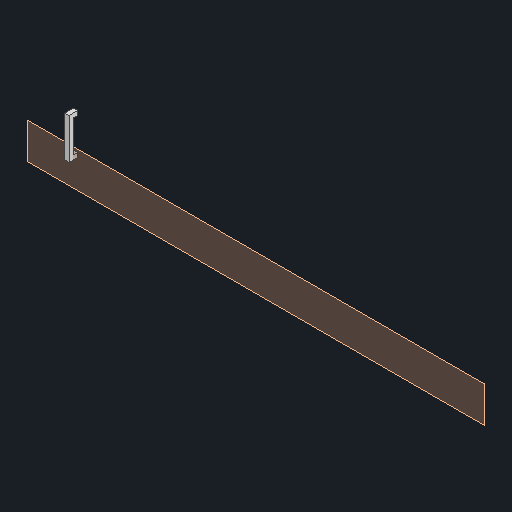
# Autodesk Inventor part: Reinforcer
Saved by Autodesk Inventor 2027 (Build 310192000, 192)
## iProperties
Created: 2026-04-15
Part Number: Reinforcer
Material: Generic
Document SubType Name: Modeling
Designer: Tueha
Density: 1 g/cm^3
Appearance: Default
Author: Tueha
Autodesk Inventor part; units mm, degrees
ref_plane "YZ Plane" through (0, 0, 0) normal (1, 0, 0) x (0, 1, 0)
ref_plane "XZ Plane" through (0, 0, 0) normal (0, 1, 0) x (-1, 0, 0)
ref_plane "XY Plane" through (0, 0, 0) normal (0, 0, 1) x (1, 0, 0)
ref_plane "Work Plane1" through (504.7277, -38.7707, -20.8442) normal (0, 0, 1) x (-1, 0, 0)
sketch "Sketch1" plane through (504.7277, -38.7707, -20.8442) normal (0, 0, 1) x (-1, 0, 0)
  line L0 (-28.8, -55.1) -> (-22.6, -55.1) projected
  line L1 (-28.8, -72) -> (-28.8, -55.1) projected
  line L2 (-28.8, -72) -> (262.8, -72) projected
  line L3 (262.8, -72) -> (262.8, -78) projected
  line L4 (262.8, -78) -> (-28.8, -78) projected
  line L5 (-28.8, -94.9) -> (-28.8, -78) projected
  line L6 (-13.3962, -94.9) -> (-28.8, -94.9) projected
  line L7 (-8.2, -97.9) -> (-13.3962, -94.9) projected
  line L8 (-8.2, -94.9) -> (-8.2, -97.9) projected
  arc A0 (-6.2, -94.9) -> (-8.2, -94.9) centre (-7.2, -94.9) ccw projected
  line L9 (-6.2, -97.9) -> (-6.2, -94.9) projected
  line L10 (-1.0038, -94.9) -> (-6.2, -97.9) projected
  line L11 (15.4038, -94.9) -> (-1.0038, -94.9) projected
  line L12 (20.6, -97.9) -> (15.4038, -94.9) projected
  line L13 (20.6, -94.9) -> (20.6, -97.9) projected
  arc A1 (22.6, -94.9) -> (20.6, -94.9) centre (21.6, -94.9) ccw projected
  line L14 (22.6, -97.9) -> (22.6, -94.9) projected
  line L15 (27.7962, -94.9) -> (22.6, -97.9) projected
  line L16 (44.2038, -94.9) -> (27.7962, -94.9) projected
  line L17 (49.4, -97.9) -> (44.2038, -94.9) projected
  line L18 (49.4, -94.9) -> (49.4, -97.9) projected
  arc A2 (51.4, -94.9) -> (49.4, -94.9) centre (50.4, -94.9) ccw projected
  line L19 (51.4, -97.9) -> (51.4, -94.9) projected
  line L20 (56.5962, -94.9) -> (51.4, -97.9) projected
  line L21 (73.0038, -94.9) -> (56.5962, -94.9) projected
  line L22 (78.2, -97.9) -> (73.0038, -94.9) projected
  line L23 (78.2, -94.9) -> (78.2, -97.9) projected
  arc A3 (80.2, -94.9) -> (78.2, -94.9) centre (79.2, -94.9) ccw projected
  line L24 (80.2, -97.9) -> (80.2, -94.9) projected
  line L25 (85.3962, -94.9) -> (80.2, -97.9) projected
  line L26 (101.8038, -94.9) -> (85.3962, -94.9) projected
  line L27 (107, -97.9) -> (101.8038, -94.9) projected
  line L28 (107, -94.9) -> (107, -97.9) projected
  arc A4 (109, -94.9) -> (107, -94.9) centre (108, -94.9) ccw projected
  line L29 (109, -97.9) -> (109, -94.9) projected
  line L30 (114.1962, -94.9) -> (109, -97.9) projected
  line L31 (130.6038, -94.9) -> (114.1962, -94.9) projected
  line L32 (135.8, -97.9) -> (130.6038, -94.9) projected
  line L33 (135.8, -94.9) -> (135.8, -97.9) projected
  arc A5 (137.8, -94.9) -> (135.8, -94.9) centre (136.8, -94.9) ccw projected
  line L34 (137.8, -97.9) -> (137.8, -94.9) projected
  line L35 (142.9962, -94.9) -> (137.8, -97.9) projected
  line L36 (159.4038, -94.9) -> (142.9962, -94.9) projected
  line L37 (164.6, -97.9) -> (159.4038, -94.9) projected
  line L38 (164.6, -94.9) -> (164.6, -97.9) projected
  arc A6 (166.6, -94.9) -> (164.6, -94.9) centre (165.6, -94.9) ccw projected
  line L39 (166.6, -97.9) -> (166.6, -94.9) projected
  line L40 (171.7962, -94.9) -> (166.6, -97.9) projected
  line L41 (188.2038, -94.9) -> (171.7962, -94.9) projected
  line L42 (193.4, -97.9) -> (188.2038, -94.9) projected
  line L43 (193.4, -94.9) -> (193.4, -97.9) projected
  arc A7 (195.4, -94.9) -> (193.4, -94.9) centre (194.4, -94.9) ccw projected
  line L44 (195.4, -97.9) -> (195.4, -94.9) projected
  line L45 (200.5962, -94.9) -> (195.4, -97.9) projected
  line L46 (217.0038, -94.9) -> (200.5962, -94.9) projected
  line L47 (222.2, -97.9) -> (217.0038, -94.9) projected
  line L48 (222.2, -94.9) -> (222.2, -97.9) projected
  arc A8 (224.2, -94.9) -> (222.2, -94.9) centre (223.2, -94.9) ccw projected
  line L49 (224.2, -97.9) -> (224.2, -94.9) projected
  line L50 (229.3962, -94.9) -> (224.2, -97.9) projected
  line L51 (245.8038, -94.9) -> (229.3962, -94.9) projected
  line L52 (251, -97.9) -> (245.8038, -94.9) projected
  line L53 (251, -94.9) -> (251, -97.9) projected
  arc A9 (253, -94.9) -> (251, -94.9) centre (252, -94.9) ccw projected
  line L54 (253, -97.9) -> (253, -94.9) projected
  line L55 (258.1962, -94.9) -> (253, -97.9) projected
  line L56 (274.6038, -94.9) -> (258.1962, -94.9) projected
  line L57 (279.8, -97.9) -> (274.6038, -94.9) projected
  line L58 (279.8, -94.9) -> (279.8, -97.9) projected
  arc A10 (281.8, -94.9) -> (279.8, -94.9) centre (280.8, -94.9) ccw projected
  line L59 (281.8, -97.9) -> (281.8, -94.9) projected
  line L60 (286.9962, -94.9) -> (281.8, -97.9) projected
  line L61 (303.4038, -94.9) -> (286.9962, -94.9) projected
  line L62 (308.6, -97.9) -> (303.4038, -94.9) projected
  line L63 (308.6, -94.9) -> (308.6, -97.9) projected
  arc A11 (310.6, -94.9) -> (308.6, -94.9) centre (309.6, -94.9) ccw projected
  line L64 (310.6, -97.9) -> (310.6, -94.9) projected
  line L65 (315.7962, -94.9) -> (310.6, -97.9) projected
  line L66 (332.2038, -94.9) -> (315.7962, -94.9) projected
  line L67 (337.4, -97.9) -> (332.2038, -94.9) projected
  line L68 (337.4, -94.9) -> (337.4, -97.9) projected
  arc A12 (339.4, -94.9) -> (337.4, -94.9) centre (338.4, -94.9) ccw projected
  line L69 (339.4, -97.9) -> (339.4, -94.9) projected
  line L70 (344.5962, -94.9) -> (339.4, -97.9) projected
  line L71 (361.0038, -94.9) -> (344.5962, -94.9) projected
  line L72 (366.2, -97.9) -> (361.0038, -94.9) projected
  line L73 (366.2, -94.9) -> (366.2, -97.9) projected
  arc A13 (368.2, -94.9) -> (366.2, -94.9) centre (367.2, -94.9) ccw projected
  line L74 (368.2, -97.9) -> (368.2, -94.9) projected
  line L75 (373.3962, -94.9) -> (368.2, -97.9) projected
  line L76 (389.8038, -94.9) -> (373.3962, -94.9) projected
  line L77 (395, -97.9) -> (389.8038, -94.9) projected
  line L78 (395, -94.9) -> (395, -97.9) projected
  arc A14 (397, -94.9) -> (395, -94.9) centre (396, -94.9) ccw projected
  line L79 (397, -97.9) -> (397, -94.9) projected
  line L80 (402.1962, -94.9) -> (397, -97.9) projected
  line L81 (418.6038, -94.9) -> (402.1962, -94.9) projected
  line L82 (423.8, -97.9) -> (418.6038, -94.9) projected
  line L83 (423.8, -94.9) -> (423.8, -97.9) projected
  arc A15 (425.8, -94.9) -> (423.8, -94.9) centre (424.8, -94.9) ccw projected
  line L84 (425.8, -97.9) -> (425.8, -94.9) projected
  line L85 (430.9962, -94.9) -> (425.8, -97.9) projected
  line L86 (447.4038, -94.9) -> (430.9962, -94.9) projected
  line L87 (452.6, -97.9) -> (447.4038, -94.9) projected
  line L88 (452.6, -94.9) -> (452.6, -97.9) projected
  arc A16 (454.6, -94.9) -> (452.6, -94.9) centre (453.6, -94.9) ccw projected
  line L89 (454.6, -97.9) -> (454.6, -94.9) projected
  line L90 (459.7962, -94.9) -> (454.6, -97.9) projected
  line L91 (476.2038, -94.9) -> (459.7962, -94.9) projected
  line L92 (481.4, -97.9) -> (476.2038, -94.9) projected
  line L93 (481.4, -94.9) -> (481.4, -97.9) projected
  arc A17 (483.4, -94.9) -> (481.4, -94.9) centre (482.4, -94.9) ccw projected
  line L94 (483.4, -97.9) -> (483.4, -94.9) projected
  line L95 (488.5962, -94.9) -> (483.4, -97.9) projected
  line L96 (505.0038, -94.9) -> (488.5962, -94.9) projected
  line L97 (510.2, -97.9) -> (505.0038, -94.9) projected
  line L98 (510.2, -94.9) -> (510.2, -97.9) projected
  arc A18 (512.2, -94.9) -> (510.2, -94.9) centre (511.2, -94.9) ccw projected
  line L99 (512.2, -97.9) -> (512.2, -94.9) projected
  line L100 (517.3962, -94.9) -> (512.2, -97.9) projected
  line L101 (533.8038, -94.9) -> (517.3962, -94.9) projected
  line L102 (539, -97.9) -> (533.8038, -94.9) projected
  line L103 (539, -94.9) -> (539, -97.9) projected
  arc A19 (541, -94.9) -> (539, -94.9) centre (540, -94.9) ccw projected
  line L104 (541, -97.9) -> (541, -94.9) projected
  line L105 (546.1962, -94.9) -> (541, -97.9) projected
  line L106 (546.1962, -94.9) -> (554.4, -94.9) projected
  line L107 (554.4, -55.1) -> (554.4, -94.9) projected
  line L108 (531.7962, -55.1) -> (554.4, -55.1) projected
  line L109 (526.6, -52.1) -> (531.7962, -55.1) projected
  line L110 (526.6, -55.1) -> (526.6, -52.1) projected
  arc A20 (524.6, -55.1) -> (526.6, -55.1) centre (525.6, -55.1) ccw projected
  line L111 (524.6, -52.1) -> (524.6, -55.1) projected
  line L112 (519.4038, -55.1) -> (524.6, -52.1) projected
  line L113 (502.9962, -55.1) -> (519.4038, -55.1) projected
  line L114 (497.8, -52.1) -> (502.9962, -55.1) projected
  line L115 (497.8, -55.1) -> (497.8, -52.1) projected
  arc A21 (495.8, -55.1) -> (497.8, -55.1) centre (496.8, -55.1) ccw projected
  line L116 (495.8, -52.1) -> (495.8, -55.1) projected
  line L117 (490.6038, -55.1) -> (495.8, -52.1) projected
  line L118 (474.1962, -55.1) -> (490.6038, -55.1) projected
  line L119 (469, -52.1) -> (474.1962, -55.1) projected
  line L120 (469, -55.1) -> (469, -52.1) projected
  arc A22 (467, -55.1) -> (469, -55.1) centre (468, -55.1) ccw projected
  line L121 (467, -52.1) -> (467, -55.1) projected
  line L122 (461.8038, -55.1) -> (467, -52.1) projected
  line L123 (445.3962, -55.1) -> (461.8038, -55.1) projected
  line L124 (440.2, -52.1) -> (445.3962, -55.1) projected
  line L125 (440.2, -55.1) -> (440.2, -52.1) projected
  arc A23 (438.2, -55.1) -> (440.2, -55.1) centre (439.2, -55.1) ccw projected
  line L126 (438.2, -52.1) -> (438.2, -55.1) projected
  line L127 (433.0038, -55.1) -> (438.2, -52.1) projected
  line L128 (416.5962, -55.1) -> (433.0038, -55.1) projected
  line L129 (411.4, -52.1) -> (416.5962, -55.1) projected
  line L130 (411.4, -55.1) -> (411.4, -52.1) projected
  arc A24 (409.4, -55.1) -> (411.4, -55.1) centre (410.4, -55.1) ccw projected
  line L131 (409.4, -52.1) -> (409.4, -55.1) projected
  line L132 (404.2038, -55.1) -> (409.4, -52.1) projected
  line L133 (387.7962, -55.1) -> (404.2038, -55.1) projected
  line L134 (382.6, -52.1) -> (387.7962, -55.1) projected
  line L135 (382.6, -55.1) -> (382.6, -52.1) projected
  arc A25 (380.6, -55.1) -> (382.6, -55.1) centre (381.6, -55.1) ccw projected
  line L136 (380.6, -52.1) -> (380.6, -55.1) projected
  line L137 (375.4038, -55.1) -> (380.6, -52.1) projected
  line L138 (358.9962, -55.1) -> (375.4038, -55.1) projected
  line L139 (353.8, -52.1) -> (358.9962, -55.1) projected
  line L140 (353.8, -55.1) -> (353.8, -52.1) projected
  arc A26 (351.8, -55.1) -> (353.8, -55.1) centre (352.8, -55.1) ccw projected
  line L141 (351.8, -52.1) -> (351.8, -55.1) projected
  line L142 (346.6038, -55.1) -> (351.8, -52.1) projected
  line L143 (330.1962, -55.1) -> (346.6038, -55.1) projected
  line L144 (325, -52.1) -> (330.1962, -55.1) projected
  line L145 (325, -55.1) -> (325, -52.1) projected
  arc A27 (323, -55.1) -> (325, -55.1) centre (324, -55.1) ccw projected
  line L146 (323, -52.1) -> (323, -55.1) projected
  line L147 (317.8038, -55.1) -> (323, -52.1) projected
  line L148 (301.3962, -55.1) -> (317.8038, -55.1) projected
  line L149 (296.2, -52.1) -> (301.3962, -55.1) projected
  line L150 (296.2, -55.1) -> (296.2, -52.1) projected
  arc A28 (294.2, -55.1) -> (296.2, -55.1) centre (295.2, -55.1) ccw projected
  line L151 (294.2, -52.1) -> (294.2, -55.1) projected
  line L152 (289.0038, -55.1) -> (294.2, -52.1) projected
  line L153 (272.5962, -55.1) -> (289.0038, -55.1) projected
  line L154 (267.4, -52.1) -> (272.5962, -55.1) projected
  line L155 (267.4, -55.1) -> (267.4, -52.1) projected
  arc A29 (265.4, -55.1) -> (267.4, -55.1) centre (266.4, -55.1) ccw projected
  line L156 (265.4, -52.1) -> (265.4, -55.1) projected
  line L157 (260.2038, -55.1) -> (265.4, -52.1) projected
  line L158 (243.7962, -55.1) -> (260.2038, -55.1) projected
  line L159 (238.6, -52.1) -> (243.7962, -55.1) projected
  line L160 (238.6, -55.1) -> (238.6, -52.1) projected
  arc A30 (236.6, -55.1) -> (238.6, -55.1) centre (237.6, -55.1) ccw projected
  line L161 (236.6, -52.1) -> (236.6, -55.1) projected
  line L162 (231.4038, -55.1) -> (236.6, -52.1) projected
  line L163 (214.9962, -55.1) -> (231.4038, -55.1) projected
  line L164 (209.8, -52.1) -> (214.9962, -55.1) projected
  line L165 (209.8, -55.1) -> (209.8, -52.1) projected
  arc A31 (207.8, -55.1) -> (209.8, -55.1) centre (208.8, -55.1) ccw projected
  line L166 (207.8, -52.1) -> (207.8, -55.1) projected
  line L167 (202.6038, -55.1) -> (207.8, -52.1) projected
  line L168 (186.1962, -55.1) -> (202.6038, -55.1) projected
  line L169 (181, -52.1) -> (186.1962, -55.1) projected
  line L170 (181, -55.1) -> (181, -52.1) projected
  arc A32 (179, -55.1) -> (181, -55.1) centre (180, -55.1) ccw projected
  line L171 (179, -52.1) -> (179, -55.1) projected
  line L172 (173.8038, -55.1) -> (179, -52.1) projected
  line L173 (157.3962, -55.1) -> (173.8038, -55.1) projected
  line L174 (152.2, -52.1) -> (157.3962, -55.1) projected
  line L175 (152.2, -55.1) -> (152.2, -52.1) projected
  arc A33 (150.2, -55.1) -> (152.2, -55.1) centre (151.2, -55.1) ccw projected
  line L176 (150.2, -52.1) -> (150.2, -55.1) projected
  line L177 (145.0038, -55.1) -> (150.2, -52.1) projected
  line L178 (128.5962, -55.1) -> (145.0038, -55.1) projected
  line L179 (123.4, -52.1) -> (128.5962, -55.1) projected
  line L180 (123.4, -55.1) -> (123.4, -52.1) projected
  arc A34 (121.4, -55.1) -> (123.4, -55.1) centre (122.4, -55.1) ccw projected
  line L181 (121.4, -52.1) -> (121.4, -55.1) projected
  line L182 (116.2038, -55.1) -> (121.4, -52.1) projected
  line L183 (99.7962, -55.1) -> (116.2038, -55.1) projected
  line L184 (94.6, -52.1) -> (99.7962, -55.1) projected
  line L185 (94.6, -55.1) -> (94.6, -52.1) projected
  arc A35 (92.6, -55.1) -> (94.6, -55.1) centre (93.6, -55.1) ccw projected
  line L186 (92.6, -52.1) -> (92.6, -55.1) projected
  line L187 (87.4038, -55.1) -> (92.6, -52.1) projected
  line L188 (70.9962, -55.1) -> (87.4038, -55.1) projected
  line L189 (65.8, -52.1) -> (70.9962, -55.1) projected
  line L190 (65.8, -55.1) -> (65.8, -52.1) projected
  arc A36 (63.8, -55.1) -> (65.8, -55.1) centre (64.8, -55.1) ccw projected
  line L191 (63.8, -52.1) -> (63.8, -55.1) projected
  line L192 (58.6038, -55.1) -> (63.8, -52.1) projected
  line L193 (42.1962, -55.1) -> (58.6038, -55.1) projected
  line L194 (37, -52.1) -> (42.1962, -55.1) projected
  line L195 (37, -55.1) -> (37, -52.1) projected
  arc A37 (35, -55.1) -> (37, -55.1) centre (36, -55.1) ccw projected
  line L196 (35, -52.1) -> (35, -55.1) projected
  line L197 (29.8038, -55.1) -> (35, -52.1) projected
  line L198 (13.3962, -55.1) -> (29.8038, -55.1) projected
  line L199 (8.2, -52.1) -> (13.3962, -55.1) projected
  line L200 (8.2, -55.1) -> (8.2, -52.1) projected
  arc A38 (6.2, -55.1) -> (8.2, -55.1) centre (7.2, -55.1) ccw projected
  line L201 (6.2, -52.1) -> (6.2, -55.1) projected
  line L202 (1.0038, -55.1) -> (6.2, -52.1) projected
  line L203 (-15.4038, -55.1) -> (1.0038, -55.1) projected
  line L204 (-20.6, -52.1) -> (-15.4038, -55.1) projected
  line L205 (-20.6, -55.1) -> (-20.6, -52.1) projected
  arc A39 (-22.6, -55.1) -> (-20.6, -55.1) centre (-21.6, -55.1) ccw projected
  line L206 (525, -66) -> (519, -66) projected
  line L207 (519, -66) -> (519, -60) projected
  line L208 (519, -60) -> (525, -60) projected
  line L209 (525, -60) -> (525, -66) projected
  line L210 (525, -84) -> (525, -90) projected
  line L211 (525, -90) -> (519, -90) projected
  line L212 (519, -90) -> (519, -84) projected
  line L213 (519, -84) -> (525, -84) projected
  line L214 (467.4, -66) -> (461.4, -66) projected
  line L215 (461.4, -66) -> (461.4, -60) projected
  line L216 (461.4, -60) -> (467.4, -60) projected
  line L217 (467.4, -60) -> (467.4, -66) projected
  line L218 (467.4, -84) -> (467.4, -90) projected
  line L219 (467.4, -90) -> (461.4, -90) projected
  line L220 (461.4, -90) -> (461.4, -84) projected
  line L221 (461.4, -84) -> (467.4, -84) projected
  line L222 (409.8, -66) -> (403.8, -66) projected
  line L223 (403.8, -66) -> (403.8, -60) projected
  line L224 (403.8, -60) -> (409.8, -60) projected
  line L225 (409.8, -60) -> (409.8, -66) projected
  line L226 (409.8, -84) -> (409.8, -90) projected
  line L227 (409.8, -90) -> (403.8, -90) projected
  line L228 (403.8, -90) -> (403.8, -84) projected
  line L229 (403.8, -84) -> (409.8, -84) projected
  line L230 (352.2, -66) -> (346.2, -66) projected
  line L231 (346.2, -66) -> (346.2, -60) projected
  line L232 (346.2, -60) -> (352.2, -60) projected
  line L233 (352.2, -60) -> (352.2, -66) projected
  line L234 (352.2, -84) -> (352.2, -90) projected
  line L235 (352.2, -90) -> (346.2, -90) projected
  line L236 (346.2, -90) -> (346.2, -84) projected
  line L237 (346.2, -84) -> (352.2, -84) projected
  line L238 (294.6, -66) -> (288.6, -66) projected
  line L239 (288.6, -66) -> (288.6, -60) projected
  line L240 (288.6, -60) -> (294.6, -60) projected
  line L241 (294.6, -60) -> (294.6, -66) projected
  line L242 (294.6, -84) -> (294.6, -90) projected
  line L243 (294.6, -90) -> (288.6, -90) projected
  line L244 (288.6, -90) -> (288.6, -84) projected
  line L245 (288.6, -84) -> (294.6, -84) projected
  line L246 (237, -66) -> (231, -66) projected
  line L247 (231, -66) -> (231, -60) projected
  line L248 (231, -60) -> (237, -60) projected
  line L249 (237, -60) -> (237, -66) projected
  line L250 (237, -84) -> (237, -90) projected
  line L251 (237, -90) -> (231, -90) projected
  line L252 (231, -90) -> (231, -84) projected
  line L253 (231, -84) -> (237, -84) projected
  line L254 (179.4, -66) -> (173.4, -66) projected
  line L255 (173.4, -66) -> (173.4, -60) projected
  line L256 (173.4, -60) -> (179.4, -60) projected
  line L257 (179.4, -60) -> (179.4, -66) projected
  line L258 (179.4, -84) -> (179.4, -90) projected
  line L259 (179.4, -90) -> (173.4, -90) projected
  line L260 (173.4, -90) -> (173.4, -84) projected
  line L261 (173.4, -84) -> (179.4, -84) projected
  line L262 (121.8, -66) -> (115.8, -66) projected
  line L263 (115.8, -66) -> (115.8, -60) projected
  line L264 (115.8, -60) -> (121.8, -60) projected
  line L265 (121.8, -60) -> (121.8, -66) projected
  line L266 (121.8, -84) -> (121.8, -90) projected
  line L267 (121.8, -90) -> (115.8, -90) projected
  line L268 (115.8, -90) -> (115.8, -84) projected
  line L269 (115.8, -84) -> (121.8, -84) projected
  line L270 (64.2, -66) -> (58.2, -66) projected
  line L271 (58.2, -66) -> (58.2, -60) projected
  line L272 (58.2, -60) -> (64.2, -60) projected
  line L273 (64.2, -60) -> (64.2, -66) projected
  line L274 (64.2, -84) -> (64.2, -90) projected
  line L275 (64.2, -90) -> (58.2, -90) projected
  line L276 (58.2, -90) -> (58.2, -84) projected
  line L277 (58.2, -84) -> (64.2, -84) projected
  line L278 (6.6, -66) -> (0.6, -66) projected
  line L279 (0.6, -66) -> (0.6, -60) projected
  line L280 (0.6, -60) -> (6.6, -60) projected
  line L281 (6.6, -60) -> (6.6, -66) projected
  line L282 (6.6, -84) -> (6.6, -90) projected
  line L283 (6.6, -90) -> (0.6, -90) projected
  line L284 (0.6, -90) -> (0.6, -84) projected
  line L285 (0.6, -84) -> (6.6, -84) projected
  line L286 (-28.8, 19.9) -> (-22.6, 19.9) projected
  line L287 (-28.8, 3) -> (-28.8, 19.9) projected
  line L288 (-28.8, 3) -> (262.8, 3) projected
  line L289 (262.8, 3) -> (262.8, -3) projected
  line L290 (262.8, -3) -> (-28.8, -3) projected
  line L291 (-28.8, -19.9) -> (-28.8, -3) projected
  line L292 (-13.3962, -19.9) -> (-28.8, -19.9) projected
  line L293 (-8.2, -22.9) -> (-13.3962, -19.9) projected
  line L294 (-8.2, -19.9) -> (-8.2, -22.9) projected
  arc A40 (-6.2, -19.9) -> (-8.2, -19.9) centre (-7.2, -19.9) ccw projected
  line L295 (-6.2, -22.9) -> (-6.2, -19.9) projected
  line L296 (-1.0038, -19.9) -> (-6.2, -22.9) projected
  line L297 (15.4038, -19.9) -> (-1.0038, -19.9) projected
  line L298 (20.6, -22.9) -> (15.4038, -19.9) projected
  line L299 (20.6, -19.9) -> (20.6, -22.9) projected
  arc A41 (22.6, -19.9) -> (20.6, -19.9) centre (21.6, -19.9) ccw projected
  line L300 (22.6, -22.9) -> (22.6, -19.9) projected
  line L301 (27.7962, -19.9) -> (22.6, -22.9) projected
  line L302 (44.2038, -19.9) -> (27.7962, -19.9) projected
  line L303 (49.4, -22.9) -> (44.2038, -19.9) projected
  line L304 (49.4, -19.9) -> (49.4, -22.9) projected
  arc A42 (51.4, -19.9) -> (49.4, -19.9) centre (50.4, -19.9) ccw projected
  line L305 (51.4, -22.9) -> (51.4, -19.9) projected
  line L306 (56.5962, -19.9) -> (51.4, -22.9) projected
  line L307 (73.0038, -19.9) -> (56.5962, -19.9) projected
  line L308 (78.2, -22.9) -> (73.0038, -19.9) projected
  line L309 (78.2, -19.9) -> (78.2, -22.9) projected
  arc A43 (80.2, -19.9) -> (78.2, -19.9) centre (79.2, -19.9) ccw projected
  line L310 (80.2, -22.9) -> (80.2, -19.9) projected
  line L311 (85.3962, -19.9) -> (80.2, -22.9) projected
  line L312 (101.8038, -19.9) -> (85.3962, -19.9) projected
  line L313 (107, -22.9) -> (101.8038, -19.9) projected
  line L314 (107, -19.9) -> (107, -22.9) projected
  arc A44 (109, -19.9) -> (107, -19.9) centre (108, -19.9) ccw projected
  line L315 (109, -22.9) -> (109, -19.9) projected
  line L316 (114.1962, -19.9) -> (109, -22.9) projected
  line L317 (130.6038, -19.9) -> (114.1962, -19.9) projected
  line L318 (135.8, -22.9) -> (130.6038, -19.9) projected
  line L319 (135.8, -19.9) -> (135.8, -22.9) projected
  arc A45 (137.8, -19.9) -> (135.8, -19.9) centre (136.8, -19.9) ccw projected
  line L320 (137.8, -22.9) -> (137.8, -19.9) projected
  line L321 (142.9962, -19.9) -> (137.8, -22.9) projected
  line L322 (159.4038, -19.9) -> (142.9962, -19.9) projected
  line L323 (164.6, -22.9) -> (159.4038, -19.9) projected
  line L324 (164.6, -19.9) -> (164.6, -22.9) projected
  arc A46 (166.6, -19.9) -> (164.6, -19.9) centre (165.6, -19.9) ccw projected
  line L325 (166.6, -22.9) -> (166.6, -19.9) projected
  line L326 (171.7962, -19.9) -> (166.6, -22.9) projected
  line L327 (188.2038, -19.9) -> (171.7962, -19.9) projected
  line L328 (193.4, -22.9) -> (188.2038, -19.9) projected
  line L329 (193.4, -19.9) -> (193.4, -22.9) projected
  arc A47 (195.4, -19.9) -> (193.4, -19.9) centre (194.4, -19.9) ccw projected
  line L330 (195.4, -22.9) -> (195.4, -19.9) projected
  line L331 (200.5962, -19.9) -> (195.4, -22.9) projected
  line L332 (217.0038, -19.9) -> (200.5962, -19.9) projected
  line L333 (222.2, -22.9) -> (217.0038, -19.9) projected
  line L334 (222.2, -19.9) -> (222.2, -22.9) projected
  arc A48 (224.2, -19.9) -> (222.2, -19.9) centre (223.2, -19.9) ccw projected
  line L335 (224.2, -22.9) -> (224.2, -19.9) projected
  line L336 (229.3962, -19.9) -> (224.2, -22.9) projected
  line L337 (245.8038, -19.9) -> (229.3962, -19.9) projected
  line L338 (251, -22.9) -> (245.8038, -19.9) projected
  line L339 (251, -19.9) -> (251, -22.9) projected
  arc A49 (253, -19.9) -> (251, -19.9) centre (252, -19.9) ccw projected
  line L340 (253, -22.9) -> (253, -19.9) projected
  line L341 (258.1962, -19.9) -> (253, -22.9) projected
  line L342 (274.6038, -19.9) -> (258.1962, -19.9) projected
  line L343 (279.8, -22.9) -> (274.6038, -19.9) projected
  line L344 (279.8, -19.9) -> (279.8, -22.9) projected
  arc A50 (281.8, -19.9) -> (279.8, -19.9) centre (280.8, -19.9) ccw projected
  line L345 (281.8, -22.9) -> (281.8, -19.9) projected
  line L346 (286.9962, -19.9) -> (281.8, -22.9) projected
  line L347 (303.4038, -19.9) -> (286.9962, -19.9) projected
  line L348 (308.6, -22.9) -> (303.4038, -19.9) projected
  line L349 (308.6, -19.9) -> (308.6, -22.9) projected
  arc A51 (310.6, -19.9) -> (308.6, -19.9) centre (309.6, -19.9) ccw projected
  line L350 (310.6, -22.9) -> (310.6, -19.9) projected
  line L351 (315.7962, -19.9) -> (310.6, -22.9) projected
  line L352 (332.2038, -19.9) -> (315.7962, -19.9) projected
  line L353 (337.4, -22.9) -> (332.2038, -19.9) projected
  line L354 (337.4, -19.9) -> (337.4, -22.9) projected
  arc A52 (339.4, -19.9) -> (337.4, -19.9) centre (338.4, -19.9) ccw projected
  line L355 (339.4, -22.9) -> (339.4, -19.9) projected
  line L356 (344.5962, -19.9) -> (339.4, -22.9) projected
  line L357 (361.0038, -19.9) -> (344.5962, -19.9) projected
  line L358 (366.2, -22.9) -> (361.0038, -19.9) projected
  line L359 (366.2, -19.9) -> (366.2, -22.9) projected
  arc A53 (368.2, -19.9) -> (366.2, -19.9) centre (367.2, -19.9) ccw projected
  line L360 (368.2, -22.9) -> (368.2, -19.9) projected
  line L361 (373.3962, -19.9) -> (368.2, -22.9) projected
  line L362 (389.8038, -19.9) -> (373.3962, -19.9) projected
  line L363 (395, -22.9) -> (389.8038, -19.9) projected
  line L364 (395, -19.9) -> (395, -22.9) projected
  arc A54 (397, -19.9) -> (395, -19.9) centre (396, -19.9) ccw projected
  line L365 (397, -22.9) -> (397, -19.9) projected
  line L366 (402.1962, -19.9) -> (397, -22.9) projected
  line L367 (418.6038, -19.9) -> (402.1962, -19.9) projected
  line L368 (423.8, -22.9) -> (418.6038, -19.9) projected
  line L369 (423.8, -19.9) -> (423.8, -22.9) projected
  arc A55 (425.8, -19.9) -> (423.8, -19.9) centre (424.8, -19.9) ccw projected
  line L370 (425.8, -22.9) -> (425.8, -19.9) projected
  line L371 (430.9962, -19.9) -> (425.8, -22.9) projected
  line L372 (447.4038, -19.9) -> (430.9962, -19.9) projected
  line L373 (452.6, -22.9) -> (447.4038, -19.9) projected
  line L374 (452.6, -19.9) -> (452.6, -22.9) projected
  arc A56 (454.6, -19.9) -> (452.6, -19.9) centre (453.6, -19.9) ccw projected
  line L375 (454.6, -22.9) -> (454.6, -19.9) projected
  line L376 (459.7962, -19.9) -> (454.6, -22.9) projected
  line L377 (476.2038, -19.9) -> (459.7962, -19.9) projected
  line L378 (481.4, -22.9) -> (476.2038, -19.9) projected
  line L379 (481.4, -19.9) -> (481.4, -22.9) projected
  arc A57 (483.4, -19.9) -> (481.4, -19.9) centre (482.4, -19.9) ccw projected
  line L380 (483.4, -22.9) -> (483.4, -19.9) projected
  line L381 (488.5962, -19.9) -> (483.4, -22.9) projected
  line L382 (505.0038, -19.9) -> (488.5962, -19.9) projected
  line L383 (510.2, -22.9) -> (505.0038, -19.9) projected
  line L384 (510.2, -19.9) -> (510.2, -22.9) projected
  arc A58 (512.2, -19.9) -> (510.2, -19.9) centre (511.2, -19.9) ccw projected
  line L385 (512.2, -22.9) -> (512.2, -19.9) projected
  line L386 (517.3962, -19.9) -> (512.2, -22.9) projected
  line L387 (533.8038, -19.9) -> (517.3962, -19.9) projected
  line L388 (539, -22.9) -> (533.8038, -19.9) projected
  line L389 (539, -19.9) -> (539, -22.9) projected
  arc A59 (541, -19.9) -> (539, -19.9) centre (540, -19.9) ccw projected
  line L390 (541, -22.9) -> (541, -19.9) projected
  line L391 (546.1962, -19.9) -> (541, -22.9) projected
  line L392 (546.1962, -19.9) -> (554.4, -19.9) projected
  line L393 (554.4, 19.9) -> (554.4, -19.9) projected
  line L394 (531.7962, 19.9) -> (554.4, 19.9) projected
  line L395 (526.6, 22.9) -> (531.7962, 19.9) projected
  line L396 (526.6, 19.9) -> (526.6, 22.9) projected
  arc A60 (524.6, 19.9) -> (526.6, 19.9) centre (525.6, 19.9) ccw projected
  line L397 (524.6, 22.9) -> (524.6, 19.9) projected
  line L398 (519.4038, 19.9) -> (524.6, 22.9) projected
  line L399 (502.9962, 19.9) -> (519.4038, 19.9) projected
  line L400 (497.8, 22.9) -> (502.9962, 19.9) projected
  line L401 (497.8, 19.9) -> (497.8, 22.9) projected
  arc A61 (495.8, 19.9) -> (497.8, 19.9) centre (496.8, 19.9) ccw projected
  line L402 (495.8, 22.9) -> (495.8, 19.9) projected
  line L403 (490.6038, 19.9) -> (495.8, 22.9) projected
  line L404 (474.1962, 19.9) -> (490.6038, 19.9) projected
  line L405 (469, 22.9) -> (474.1962, 19.9) projected
  line L406 (469, 19.9) -> (469, 22.9) projected
  arc A62 (467, 19.9) -> (469, 19.9) centre (468, 19.9) ccw projected
  line L407 (467, 22.9) -> (467, 19.9) projected
  line L408 (461.8038, 19.9) -> (467, 22.9) projected
  line L409 (445.3962, 19.9) -> (461.8038, 19.9) projected
  line L410 (440.2, 22.9) -> (445.3962, 19.9) projected
  line L411 (440.2, 19.9) -> (440.2, 22.9) projected
  arc A63 (438.2, 19.9) -> (440.2, 19.9) centre (439.2, 19.9) ccw projected
  line L412 (438.2, 22.9) -> (438.2, 19.9) projected
  line L413 (433.0038, 19.9) -> (438.2, 22.9) projected
  line L414 (416.5962, 19.9) -> (433.0038, 19.9) projected
  line L415 (411.4, 22.9) -> (416.5962, 19.9) projected
  line L416 (411.4, 19.9) -> (411.4, 22.9) projected
  arc A64 (409.4, 19.9) -> (411.4, 19.9) centre (410.4, 19.9) ccw projected
  line L417 (409.4, 22.9) -> (409.4, 19.9) projected
  line L418 (404.2038, 19.9) -> (409.4, 22.9) projected
  line L419 (387.7962, 19.9) -> (404.2038, 19.9) projected
  line L420 (382.6, 22.9) -> (387.7962, 19.9) projected
  line L421 (382.6, 19.9) -> (382.6, 22.9) projected
  arc A65 (380.6, 19.9) -> (382.6, 19.9) centre (381.6, 19.9) ccw projected
  line L422 (380.6, 22.9) -> (380.6, 19.9) projected
  line L423 (375.4038, 19.9) -> (380.6, 22.9) projected
  line L424 (358.9962, 19.9) -> (375.4038, 19.9) projected
  line L425 (353.8, 22.9) -> (358.9962, 19.9) projected
  line L426 (353.8, 19.9) -> (353.8, 22.9) projected
  arc A66 (351.8, 19.9) -> (353.8, 19.9) centre (352.8, 19.9) ccw projected
  line L427 (351.8, 22.9) -> (351.8, 19.9) projected
  line L428 (346.6038, 19.9) -> (351.8, 22.9) projected
  line L429 (330.1962, 19.9) -> (346.6038, 19.9) projected
  line L430 (325, 22.9) -> (330.1962, 19.9) projected
  line L431 (325, 19.9) -> (325, 22.9) projected
  arc A67 (323, 19.9) -> (325, 19.9) centre (324, 19.9) ccw projected
  line L432 (323, 22.9) -> (323, 19.9) projected
  line L433 (317.8038, 19.9) -> (323, 22.9) projected
  line L434 (301.3962, 19.9) -> (317.8038, 19.9) projected
  line L435 (296.2, 22.9) -> (301.3962, 19.9) projected
  line L436 (296.2, 19.9) -> (296.2, 22.9) projected
  arc A68 (294.2, 19.9) -> (296.2, 19.9) centre (295.2, 19.9) ccw projected
  line L437 (294.2, 22.9) -> (294.2, 19.9) projected
  line L438 (289.0038, 19.9) -> (294.2, 22.9) projected
  line L439 (272.5962, 19.9) -> (289.0038, 19.9) projected
  line L440 (267.4, 22.9) -> (272.5962, 19.9) projected
  line L441 (267.4, 19.9) -> (267.4, 22.9) projected
  arc A69 (265.4, 19.9) -> (267.4, 19.9) centre (266.4, 19.9) ccw projected
  line L442 (265.4, 22.9) -> (265.4, 19.9) projected
  line L443 (260.2038, 19.9) -> (265.4, 22.9) projected
  line L444 (243.7962, 19.9) -> (260.2038, 19.9) projected
  line L445 (238.6, 22.9) -> (243.7962, 19.9) projected
  line L446 (238.6, 19.9) -> (238.6, 22.9) projected
  arc A70 (236.6, 19.9) -> (238.6, 19.9) centre (237.6, 19.9) ccw projected
  line L447 (236.6, 22.9) -> (236.6, 19.9) projected
  line L448 (231.4038, 19.9) -> (236.6, 22.9) projected
  line L449 (214.9962, 19.9) -> (231.4038, 19.9) projected
  line L450 (209.8, 22.9) -> (214.9962, 19.9) projected
  line L451 (209.8, 19.9) -> (209.8, 22.9) projected
  arc A71 (207.8, 19.9) -> (209.8, 19.9) centre (208.8, 19.9) ccw projected
  line L452 (207.8, 22.9) -> (207.8, 19.9) projected
  line L453 (202.6038, 19.9) -> (207.8, 22.9) projected
  line L454 (186.1962, 19.9) -> (202.6038, 19.9) projected
  line L455 (181, 22.9) -> (186.1962, 19.9) projected
  line L456 (181, 19.9) -> (181, 22.9) projected
  arc A72 (179, 19.9) -> (181, 19.9) centre (180, 19.9) ccw projected
  line L457 (179, 22.9) -> (179, 19.9) projected
  line L458 (173.8038, 19.9) -> (179, 22.9) projected
  line L459 (157.3962, 19.9) -> (173.8038, 19.9) projected
  line L460 (152.2, 22.9) -> (157.3962, 19.9) projected
  line L461 (152.2, 19.9) -> (152.2, 22.9) projected
  arc A73 (150.2, 19.9) -> (152.2, 19.9) centre (151.2, 19.9) ccw projected
  line L462 (150.2, 22.9) -> (150.2, 19.9) projected
  line L463 (145.0038, 19.9) -> (150.2, 22.9) projected
  line L464 (128.5962, 19.9) -> (145.0038, 19.9) projected
  line L465 (123.4, 22.9) -> (128.5962, 19.9) projected
  line L466 (123.4, 19.9) -> (123.4, 22.9) projected
  arc A74 (121.4, 19.9) -> (123.4, 19.9) centre (122.4, 19.9) ccw projected
  line L467 (121.4, 22.9) -> (121.4, 19.9) projected
  line L468 (116.2038, 19.9) -> (121.4, 22.9) projected
  line L469 (99.7962, 19.9) -> (116.2038, 19.9) projected
  line L470 (94.6, 22.9) -> (99.7962, 19.9) projected
  line L471 (94.6, 19.9) -> (94.6, 22.9) projected
  arc A75 (92.6, 19.9) -> (94.6, 19.9) centre (93.6, 19.9) ccw projected
  line L472 (92.6, 22.9) -> (92.6, 19.9) projected
  line L473 (87.4038, 19.9) -> (92.6, 22.9) projected
  line L474 (70.9962, 19.9) -> (87.4038, 19.9) projected
  line L475 (65.8, 22.9) -> (70.9962, 19.9) projected
  line L476 (65.8, 19.9) -> (65.8, 22.9) projected
  arc A76 (63.8, 19.9) -> (65.8, 19.9) centre (64.8, 19.9) ccw projected
  line L477 (63.8, 22.9) -> (63.8, 19.9) projected
  line L478 (58.6038, 19.9) -> (63.8, 22.9) projected
  line L479 (42.1962, 19.9) -> (58.6038, 19.9) projected
  line L480 (37, 22.9) -> (42.1962, 19.9) projected
  line L481 (37, 19.9) -> (37, 22.9) projected
  arc A77 (35, 19.9) -> (37, 19.9) centre (36, 19.9) ccw projected
  line L482 (35, 22.9) -> (35, 19.9) projected
  line L483 (29.8038, 19.9) -> (35, 22.9) projected
  line L484 (13.3962, 19.9) -> (29.8038, 19.9) projected
  line L485 (8.2, 22.9) -> (13.3962, 19.9) projected
  line L486 (8.2, 19.9) -> (8.2, 22.9) projected
  arc A78 (6.2, 19.9) -> (8.2, 19.9) centre (7.2, 19.9) ccw projected
  line L487 (6.2, 22.9) -> (6.2, 19.9) projected
  line L488 (1.0038, 19.9) -> (6.2, 22.9) projected
  line L489 (-15.4038, 19.9) -> (1.0038, 19.9) projected
  line L490 (-20.6, 22.9) -> (-15.4038, 19.9) projected
  line L491 (-20.6, 19.9) -> (-20.6, 22.9) projected
  arc A79 (-22.6, 19.9) -> (-20.6, 19.9) centre (-21.6, 19.9) ccw projected
  line L492 (525, 9) -> (519, 9) projected
  line L493 (519, 9) -> (519, 15) projected
  line L494 (519, 15) -> (525, 15) projected
  line L495 (525, 15) -> (525, 9) projected
  line L496 (525, -9) -> (525, -15) projected
  line L497 (525, -15) -> (519, -15) projected
  line L498 (519, -15) -> (519, -9) projected
  line L499 (519, -9) -> (525, -9) projected
  line L500 (467.4, 9) -> (461.4, 9) projected
  line L501 (461.4, 9) -> (461.4, 15) projected
  line L502 (461.4, 15) -> (467.4, 15) projected
  line L503 (467.4, 15) -> (467.4, 9) projected
  line L504 (467.4, -9) -> (467.4, -15) projected
  line L505 (467.4, -15) -> (461.4, -15) projected
  line L506 (461.4, -15) -> (461.4, -9) projected
  line L507 (461.4, -9) -> (467.4, -9) projected
  line L508 (409.8, 9) -> (403.8, 9) projected
  line L509 (403.8, 9) -> (403.8, 15) projected
  line L510 (403.8, 15) -> (409.8, 15) projected
  line L511 (409.8, 15) -> (409.8, 9) projected
  line L512 (409.8, -9) -> (409.8, -15) projected
  line L513 (409.8, -15) -> (403.8, -15) projected
  line L514 (403.8, -15) -> (403.8, -9) projected
  line L515 (403.8, -9) -> (409.8, -9) projected
  line L516 (352.2, 9) -> (346.2, 9) projected
  line L517 (346.2, 9) -> (346.2, 15) projected
  line L518 (346.2, 15) -> (352.2, 15) projected
  line L519 (352.2, 15) -> (352.2, 9) projected
  line L520 (352.2, -9) -> (352.2, -15) projected
  line L521 (352.2, -15) -> (346.2, -15) projected
  line L522 (346.2, -15) -> (346.2, -9) projected
  line L523 (346.2, -9) -> (352.2, -9) projected
  line L524 (294.6, 9) -> (288.6, 9) projected
  line L525 (288.6, 9) -> (288.6, 15) projected
  line L526 (288.6, 15) -> (294.6, 15) projected
  line L527 (294.6, 15) -> (294.6, 9) projected
  line L528 (294.6, -9) -> (294.6, -15) projected
  line L529 (294.6, -15) -> (288.6, -15) projected
  line L530 (288.6, -15) -> (288.6, -9) projected
  line L531 (288.6, -9) -> (294.6, -9) projected
  line L532 (237, 9) -> (231, 9) projected
  line L533 (231, 9) -> (231, 15) projected
  line L534 (231, 15) -> (237, 15) projected
  line L535 (237, 15) -> (237, 9) projected
  line L536 (237, -9) -> (237, -15) projected
  line L537 (237, -15) -> (231, -15) projected
  line L538 (231, -15) -> (231, -9) projected
  line L539 (231, -9) -> (237, -9) projected
  line L540 (179.4, 9) -> (173.4, 9) projected
  line L541 (173.4, 9) -> (173.4, 15) projected
  line L542 (173.4, 15) -> (179.4, 15) projected
  line L543 (179.4, 15) -> (179.4, 9) projected
  line L544 (179.4, -9) -> (179.4, -15) projected
  line L545 (179.4, -15) -> (173.4, -15) projected
  line L546 (173.4, -15) -> (173.4, -9) projected
  line L547 (173.4, -9) -> (179.4, -9) projected
  line L548 (121.8, 9) -> (115.8, 9) projected
  line L549 (115.8, 9) -> (115.8, 15) projected
  line L550 (115.8, 15) -> (121.8, 15) projected
  line L551 (121.8, 15) -> (121.8, 9) projected
  line L552 (121.8, -9) -> (121.8, -15) projected
  line L553 (121.8, -15) -> (115.8, -15) projected
  line L554 (115.8, -15) -> (115.8, -9) projected
  line L555 (115.8, -9) -> (121.8, -9) projected
  line L556 (64.2, 9) -> (58.2, 9) projected
  line L557 (58.2, 9) -> (58.2, 15) projected
  line L558 (58.2, 15) -> (64.2, 15) projected
  line L559 (64.2, 15) -> (64.2, 9) projected
  line L560 (64.2, -9) -> (64.2, -15) projected
  line L561 (64.2, -15) -> (58.2, -15) projected
  line L562 (58.2, -15) -> (58.2, -9) projected
  line L563 (58.2, -9) -> (64.2, -9) projected
  line L564 (6.6, 9) -> (0.6, 9) projected
  line L565 (0.6, 9) -> (0.6, 15) projected
  line L566 (0.6, 15) -> (6.6, 15) projected
  line L567 (6.6, 15) -> (6.6, 9) projected
  line L568 (6.6, -9) -> (6.6, -15) projected
  line L569 (6.6, -15) -> (0.6, -15) projected
  line L570 (0.6, -15) -> (0.6, -9) projected
  line L571 (0.6, -9) -> (6.6, -9) projected
  point P0 (504.7277, -38.7707)
extrude "Extrusion1" add sketch "Sketch1" along normal mid plane 12 contours L206 L207 L208 L209 | L496 L497 L498 L499
sketch "Sketch2" plane through (-20.2723, -23.7707, -14.8442) normal (0, 1, 0) x (1, 0, 0)
  line L0 (0, 12) -> (0, 0) projected
  line L1 (6, 12) -> (6, 0) projected
  line L2 (0, 6) -> (6, 6)
  line L3 (6, 6) -> (6, 0)
  line L4 (6, 0) -> (0, 0)
  line L5 (0, 0) -> (0, 6)
  point P0 (20.2723, -14.8442)
  point P1 (0, 0)
  point P2 (6, 6)
  constraints: 8 end point, 2 parallel, 1 horizontal, 1 midpoint, 1 perpendicular
extrude "Extrusion2" add sketch "Sketch2" along normal up to surface (45 mm away)
body "Solid1"
